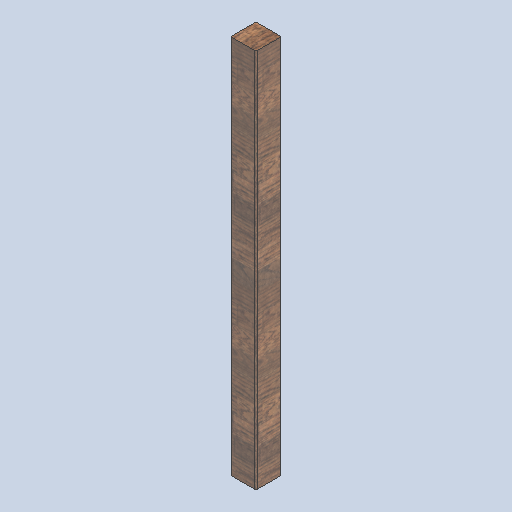
# Autodesk Inventor part: Leg
Saved by Autodesk Inventor 2022 (Build 260153000, 153)
## iProperties
Created: 2021-10-04
Part Number: Leg
Material: Generic
Document SubType Name: Modeling
Designer: Admin
Density: 1 g/cm^3
Appearance: White Ash - Java
Author: Admin
Autodesk Inventor part; units mm, degrees
ref_plane "YZ Plane" through (0, 0, 0) normal (1, 0, 0) x (0, 1, 0)
derived "Dresser SKELETON.ipt"
sketch "Base Sketch" plane through (0, 0, 0) normal (0, 1, 0) x (-1, 0, 0)
  line L0 (-635, 381) -> (635, 381) construction
  line L1 (635, 381) -> (635, -381) construction
  line L2 (635, -381) -> (-635, -381) construction
  line L3 (-635, -381) -> (-635, 381) construction
  line L4 (-635, 381) -> (635, -381) construction
  line L5 (635, 381) -> (-635, -381) construction
  line L6 (635, 381) -> (558.8, 381)
  line L7 (558.8, 381) -> (558.8, 304.8)
  line L8 (558.8, 304.8) -> (635, 304.8)
  line L9 (635, 304.8) -> (635, 381)
  line L10 (-635, 381) -> (-558.8, 381)
  line L11 (-558.8, 381) -> (-558.8, 304.8)
  line L12 (-558.8, 304.8) -> (-635, 304.8)
  line L13 (-635, 304.8) -> (-635, 381)
  line L14 (-635, -381) -> (-558.8, -381)
  line L15 (-558.8, -381) -> (-558.8, -304.8)
  line L16 (-558.8, -304.8) -> (-635, -304.8)
  line L17 (-635, -304.8) -> (-635, -381)
  line L18 (635, -381) -> (558.8, -381)
  line L19 (558.8, -381) -> (558.8, -304.8)
  line L20 (558.8, -304.8) -> (635, -304.8)
  line L21 (635, -304.8) -> (635, -381)
  point P0 (0, 0)
ref_plane "Top Plane" through (0, 1219.2, 0) normal (0, 1, 0) x (-1, 0, 0)
extrude "Extrusion1" add sketch "Base Sketch" along normal blind 1143 contours L9 L8 L7 L6
ref_plane "Mid Plane1" through (-635, 0, 342.9) normal (0, 0, 1) x (1, 0, 0)
ref_plane "Mid Plane2" through (-596.9, 0, 381) normal (1, 0, 0) x (0, 0, -1)
fillet "Fillet1" radius 3.175 4 edges at (-635, 571.5, 381) (-558.8, 571.5, 381) (-635, 571.5, 304.8) (-558.8, 571.5, 304.8)
sketch "Sketch2" plane through (-635, 0, 381) normal (0, -1, 0) x (1, 0, 0)
  line L0 (0, -76.2) -> (0, 0) projected
  line L1 (21.6803, -3.7197) -> (25.4, 0)
  line L2 (25.4, 0) -> (31.75, -6.35)
  line L3 (31.75, -6.35) -> (38.1, 0)
  line L4 (38.1, 0) -> (44.45, -6.35)
  line L5 (44.45, -6.35) -> (50.8, 0)
  line L6 (50.8, 0) -> (57.15, -6.35)
  line L7 (57.15, -6.35) -> (63.5, 0)
  line L8 (63.5, 0) -> (69.85, -6.35)
  line L9 (69.85, -6.35) -> (76.2, 0)
  line L10 (0, 0) -> (76.2, 0) projected
  arc A0 (21.6803, -3.7197) -> (3.7197, -21.6803) centre (12.7, -12.7) ccw
  line L11 (3.7197, -21.6803) -> (0, -25.4)
  line L12 (0, -76.2) -> (6.35, -69.85)
  line L13 (6.35, -69.85) -> (0, -63.5)
  line L14 (0, -76.2) -> (0, 0) projected
  line L15 (0, -63.5) -> (6.35, -57.15)
  line L16 (6.35, -57.15) -> (0, -50.8)
  line L17 (0, -50.8) -> (6.35, -44.45)
  line L18 (6.35, -44.45) -> (0, -38.1)
  line L19 (0, -38.1) -> (6.35, -31.75)
  line L20 (6.35, -31.75) -> (0, -25.4)
  point P0 (635, -381)
  point P1 (0, -38.1)
  point P2 (12.7, 0)
  point P3 (0, -63.5)
  point P4 (0, -63.5)
  point P5 (0, -38.1)
  point P6 (0, -38.1)
  point P7 (0, -12.7)
  dimension "d4" = 6.35
  dimension "d5" = 135
  dimension "d8" = 12.7
  dimension "d9" = 45
  constraints: 34 end point, 14 perpendicular, 7 point on line, 4 midpoint, 3 horizontal alignment, 3 vertical alignment, 2 point on circle, 2 tangent, 1 centre point, 1 collinear, 5 other
  measures "d4" distance from line of L8.end L10
  measures "d5" angle of L9 L10
  measures "d8" radius of A0
  measures "d9" angle of L0 L12
extrude "Elegant Extrusion" [suppressed]
fillet "Elegant Fillet" [suppressed]
equation "\"d1\" = dresserHeight - topThickness"
equation "\"dresserHeight\" = 1219.2"
equation "\"topThickness\" = 76.2"
body "Solid1"
